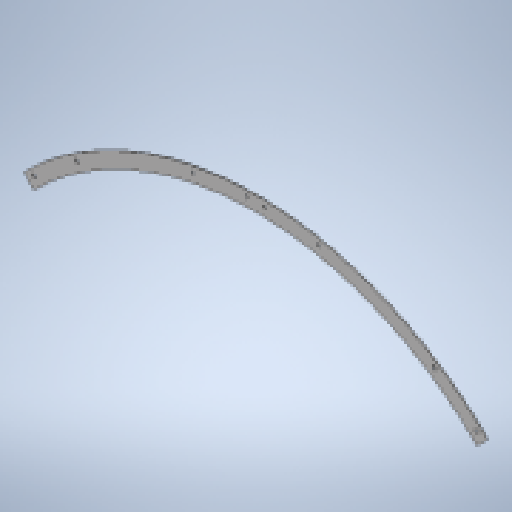
# Autodesk Inventor part: DMF2.0 01 43 Gear rim 3
Saved by Autodesk Inventor 2025 (Build 290162010, 162A)
## iProperties
Created: 2024-04-30
Part Number: DMF2.0 01 43 Gear rim 3
Material: Generic
Document SubType Name: Sheet Metal
Designer: admin
Stock Number: Барабан_Сектор_Усилителя
Density: 1 g/cm^3
Sheet Metal Rule: Default
Sheet Metal Width: 0,000 mm
Sheet Metal Length: 0,000 mm
Sheet Metal Area: 0,000 mm^2
Appearance: Default
Author: pokla
Autodesk Inventor part; units mm, degrees
ref_plane "YZ Plane" through (0, 0, 0) normal (1, 0, 0) x (0, 1, 0)
ref_plane "XZ Plane" through (0, 0, 0) normal (0, 1, 0) x (-1, 0, 0)
ref_plane "XY Plane" through (0, 0, 0) normal (0, 0, 1) x (1, 0, 0)
sketch "Sketch1" plane through (0, 0, 0) normal (0, 0, 1) x (1, 0, 0)
  circle A0 centre (0, 0) radius 650
  circle A1 centre (0, 0) radius 680
  line L0 (0, 0) -> (-480.8326, 480.8326)
  line L1 (0, 0) -> (0, 680)
  line L2 (0, 0) -> (480.8326, 480.8326)
  point P0 (-459.6194, 459.6194)
  point P1 (459.6194, 459.6194)
  dimension "d30" = 90
  dimension "d31" = 1360
  dimension "d32" = 1300
  measures "d30" angle of L2 L0
  measures "d31" diameter of A1
  measures "d32" diameter of A0
extrude "Plate1" add sketch "Sketch1" against normal blind 2 contours A0 L1 A1 L2 | L0 A1 L1 A0
sketch "Sketch2" plane through (0, 0, 0) normal (0, 0, 1) x (1, 0, 0)
  circle A0 centre (0, 0) radius 667.5
  arc A1 (480.8326, 480.8326) -> (-480.8326, 480.8326) centre (0, 0) ccw projected
  line L0 (0, 0) -> (480.8326, 480.8326) construction
  line L1 (0, 0) -> (458.5704, 485.0458) construction
  line L2 (370.8431, 555.006) -> (0, 0) construction
  line L3 (0, 0) -> (0, 667.5) construction
  line L4 (0, 0) -> (18.7209, 667.2374) construction
  line L5 (0, 0) -> (130.2228, 654.6742) construction
  line L6 (0, 0) -> (339.1403, 574.9262) construction
  line L7 (0, 0) -> (238.0449, 623.6112) construction
  dimension "d34" = 1335
  dimension "d35" = 1.607
  dimension "d36" = 9.643
  dimension "d44" = 1.607
  dimension "d45" = 9.643
  dimension "d49" = 3.214
  dimension "d50" = 9.643
  constraints: 16 end point, 1 coincident, 1 vertical, 9 other
  measures "d35" angle of L0 L1
  measures "d36" angle of L1 L2
  measures "d44" angle of L4 L3
  measures "d45" angle of L5 L4
  measures "d49" angle of L2 L6
  measures "d50" angle of L6 L7
hole "Hole1" at (458.5704, 485.0458, 0) at (370.8431, 555.006, 0) at (130.2228, 654.6742, 0) at (18.7209, 667.2374, 0) direction (0, 0, -1) diameter 8 end through all
pattern_circular "Circular Pattern1" count 2 over 45 about axis through (0, 0, -10) along (0, 0, 1) of "Hole1"
equation "\"d31\" = Колесо_диам_1"
equation "\"d32\" = Колесо_диам_2"
equation "\"d44\" = d35"
equation "\"d45\" = d36"
equation "\"d49\" = 2 * d35"
equation "\"d50\" = d36"
equation "\"d42\" = Thickness"
equation "\"d15\" = Thickness"
equation "\"BendRadius\" = Thickness"
equation "\"BendReliefWidth\" = Thickness"
equation "\"BendReliefDepth\" = 0.5 * Thickness"
equation "\"CornerReliefSize\" = 4 * Thickness"
equation "\"MinimumRemnant\" = 2 * Thickness"
equation "\"TransitionRadius\" = BendRadius"
equation "\"JacobiRadiusSize\" = BendRadius"
equation "\"GapSize\" = Thickness"
equation "\"Колесо_диам_1\" = 1360"
equation "\"Колесо_диам_2\" = 1300"
equation "\"Thickness\" = 2"
body "Solid1"
